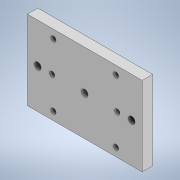
# Autodesk Inventor part: baseplate
Saved by Autodesk Inventor 2022.2 (Build 262287030, 287C)
## iProperties
Created: 2022-02-12
Part Number: baseplate
Material: Generic
Document SubType Name: Modeling
Designer: Tapendra
Density: 1 g/cm^3
Appearance: Default
Author: Tapendra
Autodesk Inventor part; units mm, degrees
ref_plane "YZ Plane" through (0, 0, 0) normal (1, 0, 0) x (0, 1, 0)
ref_plane "XZ Plane" through (0, 0, 0) normal (0, 1, 0) x (-1, 0, 0)
ref_plane "XY Plane" through (0, 0, 0) normal (0, 0, 1) x (1, 0, 0)
sketch "Sketch1" plane through (0, 0, 0) normal (0, 0, 1) x (1, 0, 0)
  line L0 (-27.5, 19) -> (27.5, 19)
  line L1 (27.5, 19) -> (27.5, -19)
  line L2 (27.5, -19) -> (-27.5, -19)
  line L3 (-27.5, -19) -> (-27.5, 19)
  line L4 (-27.5, 19) -> (27.5, -19) construction
  line L5 (27.5, 19) -> (-27.5, -19) construction
  point P0 (0, 0)
  dimension "d2" = 38
  dimension "d3" = 55
  constraints: 12 end point, 2 midpoint, 2 parallel, 1 horizontal, 1 perpendicular
  measures "d2" distance between parallel lines of L0 L2
  measures "d3" distance between parallel lines of L3 L1
extrude "Extrusion1" add sketch "Sketch1" along normal mid plane 5
sketch "Sketch2" plane through (0, 0, 2.5) normal (0, 0, 1) x (1, 0, 0)
  line L0 (-27.5, -19) -> (27.5, -19) projected
  line L1 (27.5, -19) -> (27.5, 19) projected
  line L2 (27.5, 19) -> (-27.5, 19) projected
  line L3 (-27.5, 19) -> (-27.5, -19) projected
  point P0 (0, 0)
  point P1 (-15, 15)
  point P2 (15, 15)
  point P3 (-15, -15)
  point P4 (15, -15)
  point P5 (0, 0)
  point P6 (15.6, 0)
  point P7 (-15.6, 0)
  dimension "d4" = 15
  dimension "d5" = 15
  dimension "d36" = 30
  dimension "d43" = 30
  dimension "d50" = 15.6
  dimension "d57" = 15.6
  constraints: 2 horizontal, 2 vertical, 1 coincident, 4 other
  measures "d4" horizontal distance of point (0, 0) point (-15, 15)
  measures "d5" horizontal distance of point (0, 0) point (-15, 15)
  measures "d36" distance of point (-15, 15) point (-15, -15)
  measures "d43" distance of point (15, 15) point (15, -15)
  measures "d50" distance of point (0, 0) point (15.6, 0)
  measures "d57" distance of point (0, 0) point (-15.6, 0)
hole "Hole1" at (-15.6, 0, 2.5) at (-15, 15, 2.5) at (15, 15, 2.5) at (15.6, 0, 2.5) at (15, -15, 2.5) at (-15, -15, 2.5) direction (0, 0, -1) diameter 2.5 end through all
sketch "Sketch3" plane through (0, 0, 2.5) normal (0, 0, 1) x (1, 0, 0)
  point P0 (0, 0)
  point P1 (0, 0)
  constraints: 1 coincident
hole "Hole2" at (0, 0, 2.5) direction (0, 0, -1) diameter 3.175 end through all
sketch "Sketch4" plane through (0, 0, 2.5) normal (0, 0, 1) x (1, 0, 0)
  line L0 (-27.5, 19) -> (-27.5, -19) projected
  line L1 (27.5, -19) -> (27.5, 19) projected
  point P0 (0, 0)
  point P1 (-22.5, 0)
  point P2 (22.5, 0)
  dimension "d76" = 5
  dimension "d77" = 5
  measures "d76" distance from line of L0 point (-22.5, 0)
  measures "d77" distance from line of L1 point (22.5, 0)
hole "Hole3" at (-22.5, 0, 2.5) at (22.5, 0, 2.5) direction (0, 0, -1) diameter 3.242 end through all thread size "M4x0.7" class "6H" standard "ANSI Metric M Profile"
body "Solid1"
